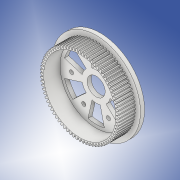
# Autodesk Inventor part: Flexspline
Saved by Autodesk Inventor 2017 SP1 (Build 210196100, 196)
## iProperties
Created: 2017-07-11
Part Number: Flexspline
Material: ABS Plastic
Document SubType Name: Modeling
Designer: zallen
Density: 1.06 g/cm^3
Appearance: CR White
Author: zallen
Autodesk Inventor part; units mm, degrees
ref_plane "YZ Plane" through (0, 0, 0) normal (1, 0, 0) x (0, 1, 0)
ref_plane "XZ Plane" through (0, 0, 0) normal (0, 1, 0) x (-1, 0, 0)
ref_plane "XY Plane" through (0, 0, 0) normal (0, 0, 1) x (1, 0, 0)
sketch "Sketch1" plane through (0, 0, 0) normal (0, 0, 1) x (1, 0, 0)
  circle A0 centre (0, 0) radius 45
  circle A1 centre (0, 0) radius 48 construction
  line L0 (0, 0) -> (52.2063, 0) construction
  arc A2 (47.9962, 0.6) -> (44.9782, 1.4) centre (42.6647, -13.4205) ccw
  arc A3 (47.9962, -0.6) -> (47.9962, 0.6) centre (28.0053, 0) ccw
  arc A4 (44.9782, -1.4) -> (47.9962, -0.6) centre (42.6647, 13.4205) ccw
  arc A5 (44.9782, -1.4) -> (44.9782, 1.4) centre (0, 0) ccw
  arc A6 (47.7828, 4.5614) -> (44.709, 5.1095) centre (43.6273, -9.8515) ccw
  arc A7 (44.9402, 2.3191) -> (47.8819, 3.3655) centre (41.4108, 16.8979) ccw
  arc A8 (47.8819, 3.3655) -> (47.7828, 4.5614) centre (27.9096, 2.3127) ccw
  circle A9 centre (0, 0) radius 45
  arc A10 (44.9402, 2.3191) -> (44.709, 5.1095) centre (0, 0) ccw
  arc A11 (47.2429, 8.4917) -> (44.1343, 8.7841) centre (44.2918, -6.2151) ccw
  arc A12 (44.5952, 6.0223) -> (47.4404, 7.3081) centre (39.8739, 20.2599) ccw
  arc A13 (47.4404, 7.3081) -> (47.2429, 8.4917) centre (27.6233, 4.6095) ccw
  circle A14 centre (0, 0) radius 45
  arc A15 (44.5952, 6.0223) -> (44.1343, 8.7841) centre (0, 0) ccw
  arc A16 (46.3803, 12.364) -> (43.2582, 12.3987) centre (44.6538, -2.5363) ccw
  arc A17 (43.9456, 9.6843) -> (46.6749, 11.2007) centre (38.0647, 23.4834) ccw
  arc A18 (46.6749, 11.2007) -> (46.3803, 12.364) centre (27.1483, 6.8749) ccw
  circle A19 centre (0, 0) radius 45
  arc A20 (43.9456, 9.6843) -> (43.2582, 12.3987) centre (0, 0) ccw
  arc A21 (45.2009, 16.1518) -> (42.0866, 15.9285) centre (44.7107, 1.1599) ccw
  arc A22 (42.9958, 13.2803) -> (45.5905, 15.0169) centre (35.9954, 26.5466) ccw
  arc A23 (45.5905, 15.0169) -> (45.2009, 16.1518) centre (26.4879, 9.0933) ccw
  circle A24 centre (0, 0) radius 45
  arc A25 (42.9958, 13.2803) -> (42.0866, 15.9285) centre (0, 0) ccw
  arc A26 (43.7127, 19.8293) -> (40.6275, 19.3496) centre (44.4622, 4.8481) ccw
  arc A27 (41.7522, 16.7855) -> (44.1947, 18.7304) centre (33.6803, 29.4284) ccw
  arc A28 (44.1947, 18.7304) -> (43.7127, 19.8293) centre (25.6465, 11.2496) ccw
  circle A29 centre (0, 0) radius 45
  arc A30 (41.7522, 16.7855) -> (40.6275, 19.3496) centre (0, 0) ccw
  arc A31 (41.9259, 23.3714) -> (38.8908, 22.6385) centre (43.91, 8.5032) ccw
  arc A32 (40.2235, 20.176) -> (42.497, 22.316) centre (31.1351, 32.1092) ccw
  arc A33 (42.497, 22.316) -> (41.9259, 23.3714) centre (24.6299, 13.329) ccw
  circle A34 centre (0, 0) radius 45
  arc A35 (40.2235, 20.176) -> (38.8908, 22.6385) centre (0, 0) ccw
  arc A36 (39.8527, 26.7538) -> (36.8885, 25.7728) centre (43.0578, 12.1002) ccw
  arc A37 (38.42, 23.4287) -> (40.509, 25.7492) centre (28.3772, 34.5706) ccw
  arc A38 (40.509, 25.7492) -> (39.8527, 26.7538) centre (23.4451, 15.3174) ccw
  circle A39 centre (0, 0) radius 45
  arc A40 (38.42, 23.4287) -> (36.8885, 25.7728) centre (0, 0) ccw
  arc A41 (37.5073, 29.9534) -> (34.6342, 28.731) centre (41.9115, 15.6145) ccw
  arc A42 (36.354, 26.5214) -> (38.2443, 29.0064) centre (25.4254, 36.7959) ccw
  arc A43 (38.2443, 29.0064) -> (37.5073, 29.9534) centre (22.1001, 17.2012) ccw
  circle A44 centre (0, 0) radius 45
  arc A45 (36.354, 26.5214) -> (34.6342, 28.731) centre (0, 0) ccw
  arc A46 (34.9056, 32.9484) -> (32.1434, 31.4929) centre (40.4789, 19.0222) ccw
  arc A47 (34.0397, 29.4329) -> (35.7184, 32.0655) centre (22.3, 38.7698) ccw
  arc A48 (35.7184, 32.0655) -> (34.9056, 32.9484) centre (20.6041, 18.9674) ccw
  circle A49 centre (0, 0) radius 45
  arc A50 (34.0397, 29.4329) -> (32.1434, 31.4929) centre (0, 0) ccw
  arc A51 (32.0655, 35.7184) -> (29.4329, 34.0397) centre (38.7698, 22.3) ccw
  arc A52 (31.4929, 32.1434) -> (32.9484, 34.9056) centre (19.0222, 40.4789) ccw
  arc A53 (32.9484, 34.9056) -> (32.0655, 35.7184) centre (18.9674, 20.6041) ccw
  circle A54 centre (0, 0) radius 45
  arc A55 (31.4929, 32.1434) -> (29.4329, 34.0397) centre (0, 0) ccw
  arc A56 (29.0064, 38.2443) -> (26.5214, 36.354) centre (36.7959, 25.4254) ccw
  arc A57 (28.731, 34.6342) -> (29.9534, 37.5073) centre (15.6145, 41.9115) ccw
  arc A58 (29.9534, 37.5073) -> (29.0064, 38.2443) centre (17.2012, 22.1001) ccw
  circle A59 centre (0, 0) radius 45
  arc A60 (28.731, 34.6342) -> (26.5214, 36.354) centre (0, 0) ccw
  arc A61 (25.7492, 40.509) -> (23.4287, 38.42) centre (34.5706, 28.3772) ccw
  arc A62 (25.7728, 36.8885) -> (26.7538, 39.8527) centre (12.1002, 43.0578) ccw
  arc A63 (26.7538, 39.8527) -> (25.7492, 40.509) centre (15.3174, 23.4451) ccw
  circle A64 centre (0, 0) radius 45
  arc A65 (25.7728, 36.8885) -> (23.4287, 38.42) centre (0, 0) ccw
  arc A66 (22.316, 42.497) -> (20.176, 40.2235) centre (32.1092, 31.1351) ccw
  arc A67 (22.6385, 38.8908) -> (23.3714, 41.9259) centre (8.5032, 43.91) ccw
  arc A68 (23.3714, 41.9259) -> (22.316, 42.497) centre (13.329, 24.6299) ccw
  circle A69 centre (0, 0) radius 45
  arc A70 (22.6385, 38.8908) -> (20.176, 40.2235) centre (0, 0) ccw
  arc A71 (18.7304, 44.1947) -> (16.7855, 41.7522) centre (29.4284, 33.6803) ccw
  arc A72 (19.3496, 40.6275) -> (19.8293, 43.7127) centre (4.8481, 44.4622) ccw
  arc A73 (19.8293, 43.7127) -> (18.7304, 44.1947) centre (11.2496, 25.6465) ccw
  circle A74 centre (0, 0) radius 45
  arc A75 (19.3496, 40.6275) -> (16.7855, 41.7522) centre (0, 0) ccw
  arc A76 (15.0169, 45.5905) -> (13.2803, 42.9958) centre (26.5466, 35.9954) ccw
  arc A77 (15.9285, 42.0866) -> (16.1518, 45.2009) centre (1.1599, 44.7107) ccw
  arc A78 (16.1518, 45.2009) -> (15.0169, 45.5905) centre (9.0933, 26.4879) ccw
  circle A79 centre (0, 0) radius 45
  arc A80 (15.9285, 42.0866) -> (13.2803, 42.9958) centre (0, 0) ccw
  arc A81 (11.2007, 46.6749) -> (9.6843, 43.9456) centre (23.4834, 38.0647) ccw
  arc A82 (12.3987, 43.2582) -> (12.364, 46.3803) centre (-2.5363, 44.6538) ccw
  arc A83 (12.364, 46.3803) -> (11.2007, 46.6749) centre (6.8749, 27.1483) ccw
  circle A84 centre (0, 0) radius 45
  arc A85 (12.3987, 43.2582) -> (9.6843, 43.9456) centre (0, 0) ccw
  arc A86 (7.3081, 47.4404) -> (6.0223, 44.5952) centre (20.2599, 39.8739) ccw
  arc A87 (8.7841, 44.1343) -> (8.4917, 47.2429) centre (-6.2151, 44.2918) ccw
  arc A88 (8.4917, 47.2429) -> (7.3081, 47.4404) centre (4.6095, 27.6233) ccw
  circle A89 centre (0, 0) radius 45
  arc A90 (8.7841, 44.1343) -> (6.0223, 44.5952) centre (0, 0) ccw
  arc A91 (3.3655, 47.8819) -> (2.3191, 44.9402) centre (16.8979, 41.4108) ccw
  arc A92 (5.1095, 44.709) -> (4.5614, 47.7828) centre (-9.8515, 43.6273) ccw
  arc A93 (4.5614, 47.7828) -> (3.3655, 47.8819) centre (2.3127, 27.9096) ccw
  circle A94 centre (0, 0) radius 45
  arc A95 (5.1095, 44.709) -> (2.3191, 44.9402) centre (0, 0) ccw
  arc A96 (-0.6, 47.9962) -> (-1.4, 44.9782) centre (13.4205, 42.6647) ccw
  arc A97 (1.4, 44.9782) -> (0.6, 47.9962) centre (-13.4205, 42.6647) ccw
  arc A98 (0.6, 47.9962) -> (-0.6, 47.9962) centre (0, 28.0053) ccw
  circle A99 centre (0, 0) radius 45
  arc A100 (1.4, 44.9782) -> (-1.4, 44.9782) centre (0, 0) ccw
  arc A101 (-4.5614, 47.7828) -> (-5.1095, 44.709) centre (9.8515, 43.6273) ccw
  arc A102 (-2.3191, 44.9402) -> (-3.3655, 47.8819) centre (-16.8979, 41.4108) ccw
  arc A103 (-3.3655, 47.8819) -> (-4.5614, 47.7828) centre (-2.3127, 27.9096) ccw
  circle A104 centre (0, 0) radius 45
  arc A105 (-2.3191, 44.9402) -> (-5.1095, 44.709) centre (0, 0) ccw
  arc A106 (-8.4917, 47.2429) -> (-8.7841, 44.1343) centre (6.2151, 44.2918) ccw
  arc A107 (-6.0223, 44.5952) -> (-7.3081, 47.4404) centre (-20.2599, 39.8739) ccw
  arc A108 (-7.3081, 47.4404) -> (-8.4917, 47.2429) centre (-4.6095, 27.6233) ccw
  circle A109 centre (0, 0) radius 45
  arc A110 (-6.0223, 44.5952) -> (-8.7841, 44.1343) centre (0, 0) ccw
  arc A111 (-12.364, 46.3803) -> (-12.3987, 43.2582) centre (2.5363, 44.6538) ccw
  arc A112 (-9.6843, 43.9456) -> (-11.2007, 46.6749) centre (-23.4834, 38.0647) ccw
  arc A113 (-11.2007, 46.6749) -> (-12.364, 46.3803) centre (-6.8749, 27.1483) ccw
  circle A114 centre (0, 0) radius 45
  arc A115 (-9.6843, 43.9456) -> (-12.3987, 43.2582) centre (0, 0) ccw
  arc A116 (-16.1518, 45.2009) -> (-15.9285, 42.0866) centre (-1.1599, 44.7107) ccw
  arc A117 (-13.2803, 42.9958) -> (-15.0169, 45.5905) centre (-26.5466, 35.9954) ccw
  arc A118 (-15.0169, 45.5905) -> (-16.1518, 45.2009) centre (-9.0933, 26.4879) ccw
  circle A119 centre (0, 0) radius 45
  arc A120 (-13.2803, 42.9958) -> (-15.9285, 42.0866) centre (0, 0) ccw
  arc A121 (-19.8293, 43.7127) -> (-19.3496, 40.6275) centre (-4.8481, 44.4622) ccw
  arc A122 (-16.7855, 41.7522) -> (-18.7304, 44.1947) centre (-29.4284, 33.6803) ccw
  arc A123 (-18.7304, 44.1947) -> (-19.8293, 43.7127) centre (-11.2496, 25.6465) ccw
  circle A124 centre (0, 0) radius 45
  arc A125 (-16.7855, 41.7522) -> (-19.3496, 40.6275) centre (0, 0) ccw
  arc A126 (-23.3714, 41.9259) -> (-22.6385, 38.8908) centre (-8.5032, 43.91) ccw
  arc A127 (-20.176, 40.2235) -> (-22.316, 42.497) centre (-32.1092, 31.1351) ccw
  arc A128 (-22.316, 42.497) -> (-23.3714, 41.9259) centre (-13.329, 24.6299) ccw
  circle A129 centre (0, 0) radius 45
  arc A130 (-20.176, 40.2235) -> (-22.6385, 38.8908) centre (0, 0) ccw
  arc A131 (-26.7538, 39.8527) -> (-25.7728, 36.8885) centre (-12.1002, 43.0578) ccw
  arc A132 (-23.4287, 38.42) -> (-25.7492, 40.509) centre (-34.5706, 28.3772) ccw
  arc A133 (-25.7492, 40.509) -> (-26.7538, 39.8527) centre (-15.3174, 23.4451) ccw
  circle A134 centre (0, 0) radius 45
  arc A135 (-23.4287, 38.42) -> (-25.7728, 36.8885) centre (0, 0) ccw
  arc A136 (-29.9534, 37.5073) -> (-28.731, 34.6342) centre (-15.6145, 41.9115) ccw
  arc A137 (-26.5214, 36.354) -> (-29.0064, 38.2443) centre (-36.7959, 25.4254) ccw
  arc A138 (-29.0064, 38.2443) -> (-29.9534, 37.5073) centre (-17.2012, 22.1001) ccw
  circle A139 centre (0, 0) radius 45
  arc A140 (-26.5214, 36.354) -> (-28.731, 34.6342) centre (0, 0) ccw
  arc A141 (-32.9484, 34.9056) -> (-31.4929, 32.1434) centre (-19.0222, 40.4789) ccw
  arc A142 (-29.4329, 34.0397) -> (-32.0655, 35.7184) centre (-38.7698, 22.3) ccw
  arc A143 (-32.0655, 35.7184) -> (-32.9484, 34.9056) centre (-18.9674, 20.6041) ccw
  circle A144 centre (0, 0) radius 45
  arc A145 (-29.4329, 34.0397) -> (-31.4929, 32.1434) centre (0, 0) ccw
  arc A146 (-35.7184, 32.0655) -> (-34.0397, 29.4329) centre (-22.3, 38.7698) ccw
  arc A147 (-32.1434, 31.4929) -> (-34.9056, 32.9484) centre (-40.4789, 19.0222) ccw
  arc A148 (-34.9056, 32.9484) -> (-35.7184, 32.0655) centre (-20.6041, 18.9674) ccw
  circle A149 centre (0, 0) radius 45
  arc A150 (-32.1434, 31.4929) -> (-34.0397, 29.4329) centre (0, 0) ccw
  arc A151 (-38.2443, 29.0064) -> (-36.354, 26.5214) centre (-25.4254, 36.7959) ccw
  arc A152 (-34.6342, 28.731) -> (-37.5073, 29.9534) centre (-41.9115, 15.6145) ccw
  arc A153 (-37.5073, 29.9534) -> (-38.2443, 29.0064) centre (-22.1001, 17.2012) ccw
  circle A154 centre (0, 0) radius 45
  arc A155 (-34.6342, 28.731) -> (-36.354, 26.5214) centre (0, 0) ccw
  arc A156 (-40.509, 25.7492) -> (-38.42, 23.4287) centre (-28.3772, 34.5706) ccw
  arc A157 (-36.8885, 25.7728) -> (-39.8527, 26.7538) centre (-43.0578, 12.1002) ccw
  arc A158 (-39.8527, 26.7538) -> (-40.509, 25.7492) centre (-23.4451, 15.3174) ccw
  circle A159 centre (0, 0) radius 45
  arc A160 (-36.8885, 25.7728) -> (-38.42, 23.4287) centre (0, 0) ccw
  arc A161 (-42.497, 22.316) -> (-40.2235, 20.176) centre (-31.1351, 32.1092) ccw
  arc A162 (-38.8908, 22.6385) -> (-41.9259, 23.3714) centre (-43.91, 8.5032) ccw
  arc A163 (-41.9259, 23.3714) -> (-42.497, 22.316) centre (-24.6299, 13.329) ccw
  circle A164 centre (0, 0) radius 45
  arc A165 (-38.8908, 22.6385) -> (-40.2235, 20.176) centre (0, 0) ccw
  arc A166 (-44.1947, 18.7304) -> (-41.7522, 16.7855) centre (-33.6803, 29.4284) ccw
  arc A167 (-40.6275, 19.3496) -> (-43.7127, 19.8293) centre (-44.4622, 4.8481) ccw
  arc A168 (-43.7127, 19.8293) -> (-44.1947, 18.7304) centre (-25.6465, 11.2496) ccw
  circle A169 centre (0, 0) radius 45
  arc A170 (-40.6275, 19.3496) -> (-41.7522, 16.7855) centre (0, 0) ccw
  arc A171 (-45.5905, 15.0169) -> (-42.9958, 13.2803) centre (-35.9954, 26.5466) ccw
  arc A172 (-42.0866, 15.9285) -> (-45.2009, 16.1518) centre (-44.7107, 1.1599) ccw
  arc A173 (-45.2009, 16.1518) -> (-45.5905, 15.0169) centre (-26.4879, 9.0933) ccw
  circle A174 centre (0, 0) radius 45
  arc A175 (-42.0866, 15.9285) -> (-42.9958, 13.2803) centre (0, 0) ccw
  arc A176 (-46.6749, 11.2007) -> (-43.9456, 9.6843) centre (-38.0647, 23.4834) ccw
  arc A177 (-43.2582, 12.3987) -> (-46.3803, 12.364) centre (-44.6538, -2.5363) ccw
  arc A178 (-46.3803, 12.364) -> (-46.6749, 11.2007) centre (-27.1483, 6.8749) ccw
  circle A179 centre (0, 0) radius 45
  arc A180 (-43.2582, 12.3987) -> (-43.9456, 9.6843) centre (0, 0) ccw
  arc A181 (-47.4404, 7.3081) -> (-44.5952, 6.0223) centre (-39.8739, 20.2599) ccw
  arc A182 (-44.1343, 8.7841) -> (-47.2429, 8.4917) centre (-44.2918, -6.2151) ccw
  arc A183 (-47.2429, 8.4917) -> (-47.4404, 7.3081) centre (-27.6233, 4.6095) ccw
  circle A184 centre (0, 0) radius 45
  arc A185 (-44.1343, 8.7841) -> (-44.5952, 6.0223) centre (0, 0) ccw
  arc A186 (-47.8819, 3.3655) -> (-44.9402, 2.3191) centre (-41.4108, 16.8979) ccw
  arc A187 (-44.709, 5.1095) -> (-47.7828, 4.5614) centre (-43.6273, -9.8515) ccw
  arc A188 (-47.7828, 4.5614) -> (-47.8819, 3.3655) centre (-27.9096, 2.3127) ccw
  circle A189 centre (0, 0) radius 45
  arc A190 (-44.709, 5.1095) -> (-44.9402, 2.3191) centre (0, 0) ccw
  arc A191 (-47.9962, -0.6) -> (-44.9782, -1.4) centre (-42.6647, 13.4205) ccw
  arc A192 (-44.9782, 1.4) -> (-47.9962, 0.6) centre (-42.6647, -13.4205) ccw
  arc A193 (-47.9962, 0.6) -> (-47.9962, -0.6) centre (-28.0053, 0) ccw
  circle A194 centre (0, 0) radius 45
  arc A195 (-44.9782, 1.4) -> (-44.9782, -1.4) centre (0, 0) ccw
  arc A196 (-47.7828, -4.5614) -> (-44.709, -5.1095) centre (-43.6273, 9.8515) ccw
  arc A197 (-44.9402, -2.3191) -> (-47.8819, -3.3655) centre (-41.4108, -16.8979) ccw
  arc A198 (-47.8819, -3.3655) -> (-47.7828, -4.5614) centre (-27.9096, -2.3127) ccw
  circle A199 centre (0, 0) radius 45
  arc A200 (-44.9402, -2.3191) -> (-44.709, -5.1095) centre (0, 0) ccw
  arc A201 (-47.2429, -8.4917) -> (-44.1343, -8.7841) centre (-44.2918, 6.2151) ccw
  arc A202 (-44.5952, -6.0223) -> (-47.4404, -7.3081) centre (-39.8739, -20.2599) ccw
  arc A203 (-47.4404, -7.3081) -> (-47.2429, -8.4917) centre (-27.6233, -4.6095) ccw
  circle A204 centre (0, 0) radius 45
  arc A205 (-44.5952, -6.0223) -> (-44.1343, -8.7841) centre (0, 0) ccw
  arc A206 (-46.3803, -12.364) -> (-43.2582, -12.3987) centre (-44.6538, 2.5363) ccw
  arc A207 (-43.9456, -9.6843) -> (-46.6749, -11.2007) centre (-38.0647, -23.4834) ccw
  arc A208 (-46.6749, -11.2007) -> (-46.3803, -12.364) centre (-27.1483, -6.8749) ccw
  circle A209 centre (0, 0) radius 45
  arc A210 (-43.9456, -9.6843) -> (-43.2582, -12.3987) centre (0, 0) ccw
  arc A211 (-45.2009, -16.1518) -> (-42.0866, -15.9285) centre (-44.7107, -1.1599) ccw
  arc A212 (-42.9958, -13.2803) -> (-45.5905, -15.0169) centre (-35.9954, -26.5466) ccw
  arc A213 (-45.5905, -15.0169) -> (-45.2009, -16.1518) centre (-26.4879, -9.0933) ccw
  circle A214 centre (0, 0) radius 45
  arc A215 (-42.9958, -13.2803) -> (-42.0866, -15.9285) centre (0, 0) ccw
  arc A216 (-43.7127, -19.8293) -> (-40.6275, -19.3496) centre (-44.4622, -4.8481) ccw
  arc A217 (-41.7522, -16.7855) -> (-44.1947, -18.7304) centre (-33.6803, -29.4284) ccw
  arc A218 (-44.1947, -18.7304) -> (-43.7127, -19.8293) centre (-25.6465, -11.2496) ccw
  circle A219 centre (0, 0) radius 45
  arc A220 (-41.7522, -16.7855) -> (-40.6275, -19.3496) centre (0, 0) ccw
  arc A221 (-41.9259, -23.3714) -> (-38.8908, -22.6385) centre (-43.91, -8.5032) ccw
  arc A222 (-40.2235, -20.176) -> (-42.497, -22.316) centre (-31.1351, -32.1092) ccw
  arc A223 (-42.497, -22.316) -> (-41.9259, -23.3714) centre (-24.6299, -13.329) ccw
  circle A224 centre (0, 0) radius 45
  arc A225 (-40.2235, -20.176) -> (-38.8908, -22.6385) centre (0, 0) ccw
  arc A226 (-39.8527, -26.7538) -> (-36.8885, -25.7728) centre (-43.0578, -12.1002) ccw
  arc A227 (-38.42, -23.4287) -> (-40.509, -25.7492) centre (-28.3772, -34.5706) ccw
  arc A228 (-40.509, -25.7492) -> (-39.8527, -26.7538) centre (-23.4451, -15.3174) ccw
  circle A229 centre (0, 0) radius 45
  arc A230 (-38.42, -23.4287) -> (-36.8885, -25.7728) centre (0, 0) ccw
  arc A231 (-37.5073, -29.9534) -> (-34.6342, -28.731) centre (-41.9115, -15.6145) ccw
  arc A232 (-36.354, -26.5214) -> (-38.2443, -29.0064) centre (-25.4254, -36.7959) ccw
  arc A233 (-38.2443, -29.0064) -> (-37.5073, -29.9534) centre (-22.1001, -17.2012) ccw
  circle A234 centre (0, 0) radius 45
  arc A235 (-36.354, -26.5214) -> (-34.6342, -28.731) centre (0, 0) ccw
  arc A236 (-34.9056, -32.9484) -> (-32.1434, -31.4929) centre (-40.4789, -19.0222) ccw
  arc A237 (-34.0397, -29.4329) -> (-35.7184, -32.0655) centre (-22.3, -38.7698) ccw
  arc A238 (-35.7184, -32.0655) -> (-34.9056, -32.9484) centre (-20.6041, -18.9674) ccw
  circle A239 centre (0, 0) radius 45
  arc A240 (-34.0397, -29.4329) -> (-32.1434, -31.4929) centre (0, 0) ccw
  arc A241 (-32.0655, -35.7184) -> (-29.4329, -34.0397) centre (-38.7698, -22.3) ccw
  arc A242 (-31.4929, -32.1434) -> (-32.9484, -34.9056) centre (-19.0222, -40.4789) ccw
  arc A243 (-32.9484, -34.9056) -> (-32.0655, -35.7184) centre (-18.9674, -20.6041) ccw
  circle A244 centre (0, 0) radius 45
  arc A245 (-31.4929, -32.1434) -> (-29.4329, -34.0397) centre (0, 0) ccw
  arc A246 (-29.0064, -38.2443) -> (-26.5214, -36.354) centre (-36.7959, -25.4254) ccw
  arc A247 (-28.731, -34.6342) -> (-29.9534, -37.5073) centre (-15.6145, -41.9115) ccw
  arc A248 (-29.9534, -37.5073) -> (-29.0064, -38.2443) centre (-17.2012, -22.1001) ccw
  circle A249 centre (0, 0) radius 45
  arc A250 (-28.731, -34.6342) -> (-26.5214, -36.354) centre (0, 0) ccw
  arc A251 (-25.7492, -40.509) -> (-23.4287, -38.42) centre (-34.5706, -28.3772) ccw
  arc A252 (-25.7728, -36.8885) -> (-26.7538, -39.8527) centre (-12.1002, -43.0578) ccw
  arc A253 (-26.7538, -39.8527) -> (-25.7492, -40.509) centre (-15.3174, -23.4451) ccw
  circle A254 centre (0, 0) radius 45
  arc A255 (-25.7728, -36.8885) -> (-23.4287, -38.42) centre (0, 0) ccw
  arc A256 (-22.316, -42.497) -> (-20.176, -40.2235) centre (-32.1092, -31.1351) ccw
  arc A257 (-22.6385, -38.8908) -> (-23.3714, -41.9259) centre (-8.5032, -43.91) ccw
  arc A258 (-23.3714, -41.9259) -> (-22.316, -42.497) centre (-13.329, -24.6299) ccw
  circle A259 centre (0, 0) radius 45
  arc A260 (-22.6385, -38.8908) -> (-20.176, -40.2235) centre (0, 0) ccw
  arc A261 (-18.7304, -44.1947) -> (-16.7855, -41.7522) centre (-29.4284, -33.6803) ccw
  arc A262 (-19.3496, -40.6275) -> (-19.8293, -43.7127) centre (-4.8481, -44.4622) ccw
  arc A263 (-19.8293, -43.7127) -> (-18.7304, -44.1947) centre (-11.2496, -25.6465) ccw
  circle A264 centre (0, 0) radius 45
  arc A265 (-19.3496, -40.6275) -> (-16.7855, -41.7522) centre (0, 0) ccw
  arc A266 (-15.0169, -45.5905) -> (-13.2803, -42.9958) centre (-26.5466, -35.9954) ccw
  arc A267 (-15.9285, -42.0866) -> (-16.1518, -45.2009) centre (-1.1599, -44.7107) ccw
  arc A268 (-16.1518, -45.2009) -> (-15.0169, -45.5905) centre (-9.0933, -26.4879) ccw
  circle A269 centre (0, 0) radius 45
  arc A270 (-15.9285, -42.0866) -> (-13.2803, -42.9958) centre (0, 0) ccw
  arc A271 (-11.2007, -46.6749) -> (-9.6843, -43.9456) centre (-23.4834, -38.0647) ccw
  arc A272 (-12.3987, -43.2582) -> (-12.364, -46.3803) centre (2.5363, -44.6538) ccw
  arc A273 (-12.364, -46.3803) -> (-11.2007, -46.6749) centre (-6.8749, -27.1483) ccw
  circle A274 centre (0, 0) radius 45
  arc A275 (-12.3987, -43.2582) -> (-9.6843, -43.9456) centre (0, 0) ccw
  arc A276 (-7.3081, -47.4404) -> (-6.0223, -44.5952) centre (-20.2599, -39.8739) ccw
  arc A277 (-8.7841, -44.1343) -> (-8.4917, -47.2429) centre (6.2151, -44.2918) ccw
  arc A278 (-8.4917, -47.2429) -> (-7.3081, -47.4404) centre (-4.6095, -27.6233) ccw
  circle A279 centre (0, 0) radius 45
  arc A280 (-8.7841, -44.1343) -> (-6.0223, -44.5952) centre (0, 0) ccw
  arc A281 (-3.3655, -47.8819) -> (-2.3191, -44.9402) centre (-16.8979, -41.4108) ccw
  arc A282 (-5.1095, -44.709) -> (-4.5614, -47.7828) centre (9.8515, -43.6273) ccw
  arc A283 (-4.5614, -47.7828) -> (-3.3655, -47.8819) centre (-2.3127, -27.9096) ccw
  circle A284 centre (0, 0) radius 45
  arc A285 (-5.1095, -44.709) -> (-2.3191, -44.9402) centre (0, 0) ccw
  arc A286 (0.6, -47.9962) -> (1.4, -44.9782) centre (-13.4205, -42.6647) ccw
  arc A287 (-1.4, -44.9782) -> (-0.6, -47.9962) centre (13.4205, -42.6647) ccw
  arc A288 (-0.6, -47.9962) -> (0.6, -47.9962) centre (0, -28.0053) ccw
  circle A289 centre (0, 0) radius 45
  arc A290 (-1.4, -44.9782) -> (1.4, -44.9782) centre (0, 0) ccw
  arc A291 (4.5614, -47.7828) -> (5.1095, -44.709) centre (-9.8515, -43.6273) ccw
  arc A292 (2.3191, -44.9402) -> (3.3655, -47.8819) centre (16.8979, -41.4108) ccw
  arc A293 (3.3655, -47.8819) -> (4.5614, -47.7828) centre (2.3127, -27.9096) ccw
  circle A294 centre (0, 0) radius 45
  arc A295 (2.3191, -44.9402) -> (5.1095, -44.709) centre (0, 0) ccw
  arc A296 (8.4917, -47.2429) -> (8.7841, -44.1343) centre (-6.2151, -44.2918) ccw
  arc A297 (6.0223, -44.5952) -> (7.3081, -47.4404) centre (20.2599, -39.8739) ccw
  arc A298 (7.3081, -47.4404) -> (8.4917, -47.2429) centre (4.6095, -27.6233) ccw
  circle A299 centre (0, 0) radius 45
  arc A300 (6.0223, -44.5952) -> (8.7841, -44.1343) centre (0, 0) ccw
  arc A301 (12.364, -46.3803) -> (12.3987, -43.2582) centre (-2.5363, -44.6538) ccw
  arc A302 (9.6843, -43.9456) -> (11.2007, -46.6749) centre (23.4834, -38.0647) ccw
  arc A303 (11.2007, -46.6749) -> (12.364, -46.3803) centre (6.8749, -27.1483) ccw
  circle A304 centre (0, 0) radius 45
  arc A305 (9.6843, -43.9456) -> (12.3987, -43.2582) centre (0, 0) ccw
  arc A306 (16.1518, -45.2009) -> (15.9285, -42.0866) centre (1.1599, -44.7107) ccw
  arc A307 (13.2803, -42.9958) -> (15.0169, -45.5905) centre (26.5466, -35.9954) ccw
  arc A308 (15.0169, -45.5905) -> (16.1518, -45.2009) centre (9.0933, -26.4879) ccw
  circle A309 centre (0, 0) radius 45
  arc A310 (13.2803, -42.9958) -> (15.9285, -42.0866) centre (0, 0) ccw
  arc A311 (19.8293, -43.7127) -> (19.3496, -40.6275) centre (4.8481, -44.4622) ccw
  arc A312 (16.7855, -41.7522) -> (18.7304, -44.1947) centre (29.4284, -33.6803) ccw
  arc A313 (18.7304, -44.1947) -> (19.8293, -43.7127) centre (11.2496, -25.6465) ccw
  circle A314 centre (0, 0) radius 45
  arc A315 (16.7855, -41.7522) -> (19.3496, -40.6275) centre (0, 0) ccw
  arc A316 (23.3714, -41.9259) -> (22.6385, -38.8908) centre (8.5032, -43.91) ccw
  arc A317 (20.176, -40.2235) -> (22.316, -42.497) centre (32.1092, -31.1351) ccw
  arc A318 (22.316, -42.497) -> (23.3714, -41.9259) centre (13.329, -24.6299) ccw
  circle A319 centre (0, 0) radius 45
  arc A320 (20.176, -40.2235) -> (22.6385, -38.8908) centre (0, 0) ccw
  arc A321 (26.7538, -39.8527) -> (25.7728, -36.8885) centre (12.1002, -43.0578) ccw
  arc A322 (23.4287, -38.42) -> (25.7492, -40.509) centre (34.5706, -28.3772) ccw
  arc A323 (25.7492, -40.509) -> (26.7538, -39.8527) centre (15.3174, -23.4451) ccw
  circle A324 centre (0, 0) radius 45
  arc A325 (23.4287, -38.42) -> (25.7728, -36.8885) centre (0, 0) ccw
  arc A326 (29.9534, -37.5073) -> (28.731, -34.6342) centre (15.6145, -41.9115) ccw
  arc A327 (26.5214, -36.354) -> (29.0064, -38.2443) centre (36.7959, -25.4254) ccw
  arc A328 (29.0064, -38.2443) -> (29.9534, -37.5073) centre (17.2012, -22.1001) ccw
  circle A329 centre (0, 0) radius 45
  arc A330 (26.5214, -36.354) -> (28.731, -34.6342) centre (0, 0) ccw
  arc A331 (32.9484, -34.9056) -> (31.4929, -32.1434) centre (19.0222, -40.4789) ccw
  arc A332 (29.4329, -34.0397) -> (32.0655, -35.7184) centre (38.7698, -22.3) ccw
  arc A333 (32.0655, -35.7184) -> (32.9484, -34.9056) centre (18.9674, -20.6041) ccw
  circle A334 centre (0, 0) radius 45
  arc A335 (29.4329, -34.0397) -> (31.4929, -32.1434) centre (0, 0) ccw
  arc A336 (35.7184, -32.0655) -> (34.0397, -29.4329) centre (22.3, -38.7698) ccw
  arc A337 (32.1434, -31.4929) -> (34.9056, -32.9484) centre (40.4789, -19.0222) ccw
  arc A338 (34.9056, -32.9484) -> (35.7184, -32.0655) centre (20.6041, -18.9674) ccw
  circle A339 centre (0, 0) radius 45
  arc A340 (32.1434, -31.4929) -> (34.0397, -29.4329) centre (0, 0) ccw
  arc A341 (38.2443, -29.0064) -> (36.354, -26.5214) centre (25.4254, -36.7959) ccw
  arc A342 (34.6342, -28.731) -> (37.5073, -29.9534) centre (41.9115, -15.6145) ccw
  arc A343 (37.5073, -29.9534) -> (38.2443, -29.0064) centre (22.1001, -17.2012) ccw
  circle A344 centre (0, 0) radius 45
  arc A345 (34.6342, -28.731) -> (36.354, -26.5214) centre (0, 0) ccw
  arc A346 (40.509, -25.7492) -> (38.42, -23.4287) centre (28.3772, -34.5706) ccw
  arc A347 (36.8885, -25.7728) -> (39.8527, -26.7538) centre (43.0578, -12.1002) ccw
  arc A348 (39.8527, -26.7538) -> (40.509, -25.7492) centre (23.4451, -15.3174) ccw
  circle A349 centre (0, 0) radius 45
  arc A350 (36.8885, -25.7728) -> (38.42, -23.4287) centre (0, 0) ccw
  arc A351 (42.497, -22.316) -> (40.2235, -20.176) centre (31.1351, -32.1092) ccw
  arc A352 (38.8908, -22.6385) -> (41.9259, -23.3714) centre (43.91, -8.5032) ccw
  arc A353 (41.9259, -23.3714) -> (42.497, -22.316) centre (24.6299, -13.329) ccw
  circle A354 centre (0, 0) radius 45
  arc A355 (38.8908, -22.6385) -> (40.2235, -20.176) centre (0, 0) ccw
  arc A356 (44.1947, -18.7304) -> (41.7522, -16.7855) centre (33.6803, -29.4284) ccw
  arc A357 (40.6275, -19.3496) -> (43.7127, -19.8293) centre (44.4622, -4.8481) ccw
  arc A358 (43.7127, -19.8293) -> (44.1947, -18.7304) centre (25.6465, -11.2496) ccw
  circle A359 centre (0, 0) radius 45
  arc A360 (40.6275, -19.3496) -> (41.7522, -16.7855) centre (0, 0) ccw
  arc A361 (45.5905, -15.0169) -> (42.9958, -13.2803) centre (35.9954, -26.5466) ccw
  arc A362 (42.0866, -15.9285) -> (45.2009, -16.1518) centre (44.7107, -1.1599) ccw
  arc A363 (45.2009, -16.1518) -> (45.5905, -15.0169) centre (26.4879, -9.0933) ccw
  circle A364 centre (0, 0) radius 45
  arc A365 (42.0866, -15.9285) -> (42.9958, -13.2803) centre (0, 0) ccw
  arc A366 (46.6749, -11.2007) -> (43.9456, -9.6843) centre (38.0647, -23.4834) ccw
  arc A367 (43.2582, -12.3987) -> (46.3803, -12.364) centre (44.6538, 2.5363) ccw
  arc A368 (46.3803, -12.364) -> (46.6749, -11.2007) centre (27.1483, -6.8749) ccw
  circle A369 centre (0, 0) radius 45
  arc A370 (43.2582, -12.3987) -> (43.9456, -9.6843) centre (0, 0) ccw
  arc A371 (47.4404, -7.3081) -> (44.5952, -6.0223) centre (39.8739, -20.2599) ccw
  arc A372 (44.1343, -8.7841) -> (47.2429, -8.4917) centre (44.2918, 6.2151) ccw
  arc A373 (47.2429, -8.4917) -> (47.4404, -7.3081) centre (27.6233, -4.6095) ccw
  circle A374 centre (0, 0) radius 45
  arc A375 (44.1343, -8.7841) -> (44.5952, -6.0223) centre (0, 0) ccw
  arc A376 (47.8819, -3.3655) -> (44.9402, -2.3191) centre (41.4108, -16.8979) ccw
  arc A377 (44.709, -5.1095) -> (47.7828, -4.5614) centre (43.6273, 9.8515) ccw
  arc A378 (47.7828, -4.5614) -> (47.8819, -3.3655) centre (27.9096, -2.3127) ccw
  circle A379 centre (0, 0) radius 45
  arc A380 (44.709, -5.1095) -> (44.9402, -2.3191) centre (0, 0) ccw
  point P0 (48.0053, 0)
  point P1 (47.8413, 3.9642)
  point P2 (47.3505, 7.9014)
  point P3 (46.5363, 11.7846)
  point P4 (45.4042, 15.5873)
  point P5 (43.9619, 19.2835)
  point P6 (42.2194, 22.848)
  point P7 (40.1884, 26.2564)
  point P8 (37.8829, 29.4854)
  point P9 (35.3186, 32.5131)
  point P10 (32.5131, 35.3186)
  point P11 (29.4854, 37.8829)
  point P12 (26.2564, 40.1884)
  point P13 (22.848, 42.2194)
  point P14 (19.2835, 43.9619)
  point P15 (15.5873, 45.4042)
  point P16 (11.7846, 46.5363)
  point P17 (7.9014, 47.3505)
  point P18 (3.9642, 47.8413)
  point P19 (0, 48.0053)
  point P20 (-3.9642, 47.8413)
  point P21 (-7.9014, 47.3505)
  point P22 (-11.7846, 46.5363)
  point P23 (-15.5873, 45.4042)
  point P24 (-19.2835, 43.9619)
  point P25 (-22.848, 42.2194)
  point P26 (-26.2564, 40.1884)
  point P27 (-29.4854, 37.8829)
  point P28 (-32.5131, 35.3186)
  point P29 (-35.3186, 32.5131)
  point P30 (-37.8829, 29.4854)
  point P31 (-40.1884, 26.2564)
  point P32 (-42.2194, 22.848)
  point P33 (-43.9619, 19.2835)
  point P34 (-45.4042, 15.5873)
  point P35 (-46.5363, 11.7846)
  point P36 (-47.3505, 7.9014)
  point P37 (-47.8413, 3.9642)
  point P38 (-48.0053, 0)
  point P39 (-47.8413, -3.9642)
  point P40 (-47.3505, -7.9014)
  point P41 (-46.5363, -11.7846)
  point P42 (-45.4042, -15.5873)
  point P43 (-43.9619, -19.2835)
  point P44 (-42.2194, -22.848)
  point P45 (-40.1884, -26.2564)
  point P46 (-37.8829, -29.4854)
  point P47 (-35.3186, -32.5131)
  point P48 (-32.5131, -35.3186)
  point P49 (-29.4854, -37.8829)
  point P50 (-26.2564, -40.1884)
  point P51 (-22.848, -42.2194)
  point P52 (-19.2835, -43.9619)
  point P53 (-15.5873, -45.4042)
  point P54 (-11.7846, -46.5363)
  point P55 (-7.9014, -47.3505)
  point P56 (-3.9642, -47.8413)
  point P57 (0, -48.0053)
  point P58 (3.9642, -47.8413)
  point P59 (7.9014, -47.3505)
  point P60 (11.7846, -46.5363)
  point P61 (15.5873, -45.4042)
  point P62 (19.2835, -43.9619)
  point P63 (22.848, -42.2194)
  point P64 (26.2564, -40.1884)
  point P65 (29.4854, -37.8829)
  point P66 (32.5131, -35.3186)
  point P67 (35.3186, -32.5131)
  point P68 (37.8829, -29.4854)
  point P69 (40.1884, -26.2564)
  point P70 (42.2194, -22.848)
  point P71 (43.9619, -19.2835)
  point P72 (45.4042, -15.5873)
  point P73 (46.5363, -11.7846)
  point P74 (47.3505, -7.9014)
  point P75 (47.8413, -3.9642)
  dimension "d2" = 15
  dimension "d3" = 20
  dimension "d4" = 1.2
  dimension "d5" = 1.4
  dimension "d6" = 3
  dimension "d9" = 360
  constraints: 611 point on circle, 305 centre point, 2 coincident, 2 end point, 2 symmetric about line, 1 horizontal, 1 point on line, 1446 other
  measures "d2" radius of A2
  measures "d3" radius of A3
  measures "d4" distance of A1.end A1.start
  measures "d5" distance from line of L0 A2.end
extrude "Extrusion1" add sketch "Sketch1" along normal blind 20
sketch "Sketch2" plane through (0, 0, 20) normal (0, 0, 1) x (1, 0, 0)
  circle A0 centre (0, 0) radius 44
  dimension "d13" = 88
  constraints: 1 centre point, 1 coincident
  measures "d13" diameter of A0
extrude "Extrusion2" cut sketch "Sketch2" against normal through all
sketch "Sketch3" plane through (0, 0, 0) normal (0, 0, -1) x (-1, 0, 0)
  circle A0 centre (0, 0) radius 11
  circle A1 centre (0, 0) radius 17.5 construction
  circle A2 centre (0, 0) radius 40 construction
  circle A3 centre (0, 0) radius 54
  line L0 (-10, 38.7298) -> (-5, 16.7705)
  line L1 (10, 38.7298) -> (5, 16.7705)
  arc A4 (10, 38.7298) -> (-10, 38.7298) centre (0, 0) ccw
  arc A5 (5, 16.7705) -> (-5, 16.7705) centre (0, 0) ccw
  circle A6 centre (0, 0) radius 30 construction
  line L2 (7.7787, 28.974) -> (21.2029, 21.2235) construction
  line L3 (14.4908, 25.0988) -> (15, 25.9808) construction
  circle A7 centre (15, 25.9808) radius 2.5
  circle A8 centre (-15, 25.9808) radius 2.5
  circle A9 centre (-30, 0) radius 2.5
  circle A10 centre (-15, -25.9808) radius 2.5
  circle A11 centre (15, -25.9808) radius 2.5
  circle A12 centre (30, 0) radius 2.5
  arc A13 (-28.541, 28.0252) -> (-38.541, 10.7047) centre (0, 0) ccw
  line L4 (-28.541, 28.0252) -> (-12.0237, 12.7154)
  line L5 (-38.541, 10.7047) -> (-17.0237, 4.0551)
  arc A14 (-12.0237, 12.7154) -> (-17.0237, 4.0551) centre (0, 0) ccw
  arc A15 (-38.541, -10.7047) -> (-28.541, -28.0252) centre (0, 0) ccw
  line L6 (-38.541, -10.7047) -> (-17.0237, -4.0551)
  line L7 (-28.541, -28.0252) -> (-12.0237, -12.7154)
  arc A16 (-17.0237, -4.0551) -> (-12.0237, -12.7154) centre (0, 0) ccw
  arc A17 (-10, -38.7298) -> (10, -38.7298) centre (0, 0) ccw
  line L8 (-10, -38.7298) -> (-5, -16.7705)
  line L9 (10, -38.7298) -> (5, -16.7705)
  arc A18 (-5, -16.7705) -> (5, -16.7705) centre (0, 0) ccw
  arc A19 (28.541, -28.0252) -> (38.541, -10.7047) centre (0, 0) ccw
  line L10 (28.541, -28.0252) -> (12.0237, -12.7154)
  line L11 (38.541, -10.7047) -> (17.0237, -4.0551)
  arc A20 (12.0237, -12.7154) -> (17.0237, -4.0551) centre (0, 0) ccw
  arc A21 (38.541, 10.7047) -> (28.541, 28.0252) centre (0, 0) ccw
  line L12 (38.541, 10.7047) -> (17.0237, 4.0551)
  line L13 (28.541, 28.0252) -> (12.0237, 12.7154)
  arc A22 (17.0237, 4.0551) -> (12.0237, 12.7154) centre (0, 0) ccw
  point P0 (-21.2029, 21.2235)
  point P1 (-28.9815, -7.7505)
  point P2 (-7.7787, -28.974)
  point P3 (21.2029, -21.2235)
  point P4 (28.9815, 7.7505)
  dimension "d16" = 22
  dimension "d17" = 35
  dimension "d18" = 80
  dimension "d19" = 108
  dimension "d20" = 10
  dimension "d21" = 5
  dimension "d22" = 10
  dimension "d23" = 5
  dimension "d28" = 60
  dimension "d29" = 5
  dimension "d32" = 360
  dimension "d38" = 360
  constraints: 31 point on circle, 28 end point, 23 centre point, 7 point on line, 5 coincident, 3 concentric, 1 midpoint, 1 perpendicular, 80 other
  measures "d16" diameter of A0
  measures "d17" diameter of A1
  measures "d18" diameter of A2
  measures "d19" diameter of A3
  measures "d20" horizontal distance of point (0, 0) L0.start
  measures "d21" horizontal distance of point (0, 0) L0.end
  measures "d22" horizontal distance of point (0, 0) L1.start
  measures "d23" horizontal distance of point (0, 0) L1.end
  measures "d28" diameter of A6
  measures "d29" diameter of A7
extrude "Extrusion4" add sketch "Sketch3" along normal blind 5
body "Solid1"
